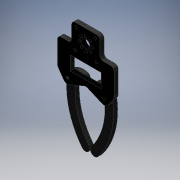
# Autodesk Inventor part: Claw
Saved by Autodesk Inventor 2016 (Build 200138000, 138)
## iProperties
Created: 2015-10-23
Part Number: Claw
Material: Generic
Document SubType Name: Modeling
Designer: alex
Density: 1 g/cm^3
Appearance: Default
Mass: 38.2404 g
Surface Area: 180.646 cm^2
Volume: 38.2404 cm^3
Author: alex
Autodesk Inventor part; units mm, degrees
ref_plane "YZ Plane" through (0, 0, 0) normal (1, 0, 0) x (0, 1, 0)
ref_plane "XZ Plane" through (0, 0, 0) normal (0, 1, 0) x (-1, 0, 0)
ref_plane "XY Plane" through (0, 0, 0) normal (0, 0, 1) x (1, 0, 0)
sketch "Sketch1" plane through (0, 0, 0) normal (0, 1, 0) x (-1, 0, 0)
  line L0 (-20, 14) -> (20, 14)
  line L1 (20, 14) -> (20, -14)
  line L2 (20, -14) -> (-20, -14)
  line L3 (-20, -14) -> (-20, 14)
  line L4 (-20, 14) -> (20, -14) construction
  line L5 (20, 14) -> (-20, -14) construction
  line L6 (-40, -52) -> (40, -52)
  line L7 (40, -52) -> (40, -14)
  line L8 (40, -14) -> (-40, -14)
  line L9 (-40, -14) -> (-40, -52)
  line L10 (-40, -52) -> (40, -14) construction
  line L11 (40, -52) -> (-40, -14) construction
  line L12 (40, -52) -> (28.303, -68.705)
  line L13 (28.303, -68.705) -> (0, -56.6911)
  line L14 (0, -33) -> (0, -82.4656)
  line L15 (-40, -52) -> (-28.303, -68.705)
  line L16 (-28.303, -68.705) -> (0, -56.6911)
  point P0 (0, 0)
  dimension "d0" = 40
  dimension "d1" = 28
  dimension "d2" = 80
  dimension "d3" = 0
  dimension "d4" = 38
  dimension "d5" = 20
  dimension "d6" = 55
  dimension "d7" = 102
  dimension "d8" = 52.1844
  dimension "d9" = 40
  constraints: 34 end point, 4 midpoint, 4 parallel, 2 horizontal, 2 perpendicular, 1 symmetric about line, 1 vertical
  measures "d0" distance of L1.end L2.end
  measures "d1" distance between parallel lines of L2 L0
  measures "d2" distance of L8.end L7.end
  measures "d3" distance between parallel lines of L2 L8
  measures "d4" distance of L6.end L7.end
  measures "d5" distance between parallel lines of L7 L1
  measures "d6" angle of L6 L12
  measures "d7" angle of L13 L12
  measures "d8" distance from line of point (0, 0) L13
  measures "d9" distance from line of L13.end L7
extrude "Extrusion1" add sketch "Sketch1" along normal blind 6
fillet "Fillet1" radius 6 3 edges at (-28.303, 3, -68.705) (28.303, 3, -68.705) (0, 3, -56.6911)
fillet "Fillet2" radius 6 2 edges at (40, 3, -52) (-40, 3, -52)
fillet "Fillet3" radius 5 2 edges at (-40, 3, -14) (40, 3, -14)
fillet "Fillet4" radius 5 2 edges at (-20, 3, -14) (20, 3, -14)
fillet "Fillet5" radius 5 2 edges at (20, 3, 14) (-20, 3, 14)
sketch "Sketch2" plane through (0, 0, 0) normal (0, -1, 0) x (1, 0, 0)
  circle A0 centre (0, -5) radius 6
  line L0 (-15, 14) -> (15, 14) projected
  circle A1 centre (-9, -5.3938) radius 2
  circle A2 centre (-6.0855, -11.6424) radius 2
  circle A3 centre (0.3938, -14) radius 2
  circle A4 centre (6.6424, -11.0855) radius 2
  circle A5 centre (9, -4.6062) radius 2
  circle A6 centre (6.0855, 1.6424) radius 2
  circle A7 centre (-0.3938, 4) radius 2
  circle A8 centre (-6.6424, 1.0855) radius 2
  line L1 (-20, 9) -> (-20, -9) projected
  circle A9 centre (13.5, 8.5) radius 2
  circle A10 centre (-13.5, 8.5) radius 2
  circle A11 centre (15, -20) radius 2
  circle A12 centre (-15, -20) radius 2
  line L2 (20, -9) -> (20, 9) projected
  line L3 (22, -29.2092) -> (-22, -29.2092)
  line L4 (-22, -29.2092) -> (-22, -49.2092)
  line L5 (-22, -49.2092) -> (22, -49.2092)
  line L6 (22, -49.2092) -> (22, -29.2092)
  line L7 (-40, -50.1082) -> (-40, -19) projected
  arc A13 (2.3444, -57.6862) -> (-2.3444, -57.6862) centre (0, -63.2092) ccw projected
  point P0 (0, 0)
  dimension "d17" = 12
  dimension "d18" = 19
  dimension "d19" = 4
  dimension "d22" = 360
  dimension "d24" = 9
  dimension "d25" = 20
  dimension "d26" = 6.6424
  dimension "d29" = 4
  dimension "d35" = 4
  dimension "d36" = 4
  dimension "d37" = 4
  dimension "d40" = 5
  dimension "d41" = 34
  dimension "d42" = 5
  dimension "d43" = 34
  dimension "d44" = 20
  dimension "d45" = 44
  dimension "d46" = 18
  dimension "d47" = 14
  dimension "d72" = 13.5
  dimension "d73" = 13.5
  dimension "d74" = 13.5
  dimension "d75" = 13.5
  constraints: 13 centre point, 8 end point, 2 parallel, 1 horizontal, 1 perpendicular, 17 other
  measures "d17" diameter of A0
  measures "d18" distance from line of L0 A0.centre
  measures "d19" diameter of A1
  measures "d24" horizontal distance of A0.centre A1.centre
  measures "d25" distance from line of L1 A0.centre
  measures "d26" horizontal distance of A0.centre A8.centre
  measures "d29" diameter of A9
  measures "d35" diameter of A10
  measures "d36" diameter of A11
  measures "d37" diameter of A12
  measures "d40" distance from line of L1 A12.centre
  measures "d41" distance from line of L0 A12.centre
  measures "d42" distance from line of L2 A11.centre
  measures "d43" distance from line of L0 A11.centre
  measures "d44" distance between parallel lines of L5 L3
  measures "d45" distance between parallel lines of L4 L6
  measures "d46" distance between parallel lines of L7 L4
  measures "d47" distance from line of A13.centre L5
  measures "d72" horizontal distance of A0.centre A9.centre
  measures "d73" horizontal distance of A0.centre A9.centre
  measures "d74" horizontal distance of A0.centre A10.centre
  measures "d75" horizontal distance of A10.centre A0.centre
extrude "holes" cut sketch "Sketch2" against normal through all
sketch "Sketch3" plane through (0, 0, 0) normal (0, -1, 0) x (1, 0, 0)
  circle A0 centre (26, -59.2092) radius 2
  circle A1 centre (-26, -59.2092) radius 2
  line L0 (22, -29.2092) -> (22, -49.2092) projected
  line L1 (-22, -49.2092) -> (22, -49.2092) projected
  line L2 (-22, -49.2092) -> (-22, -29.2092) projected
  point P0 (0, 0)
  dimension "d48" = 4
  dimension "d49" = 4
  dimension "d50" = 4
  dimension "d51" = 10
  dimension "d52" = 10
  dimension "d53" = 4
  constraints: 2 centre point
  measures "d48" diameter of A0
  measures "d49" diameter of A1
  measures "d50" distance from line of L0 A0.centre
  measures "d51" distance from line of L1 A0.centre
  measures "d52" distance from line of L1 A1.centre
  measures "d53" distance from line of L2 A1.centre
extrude "Extrusion3" cut sketch "Sketch3" against normal through all
sketch "Sketch4" plane through (0, 6, 0) normal (0, 1, 0) x (1, 0, 0)
  line L0 (0, 5.2258) -> (0, 78.3364)
  line L1 (40, 19) -> (40, 50.1082) projected
  arc A0 (25.7862, 59.4415) -> (6.4564, 137.007) centre (-72.0839, 76.243) ccw construction
  arc A1 (31.6836, 58.4291) -> (11.189, 140.6685) centre (-72.0839, 76.243) ccw
  arc A2 (19.8888, 60.454) -> (1.7238, 133.3455) centre (-72.0839, 76.243) ccw
  arc A3 (19.8888, 60.454) -> (31.6836, 58.4291) centre (25.7862, 59.4415) ccw
  arc A4 (11.189, 140.6685) -> (1.7238, 133.3455) centre (6.4564, 137.007) ccw
  arc A5 (-11.189, 140.6685) -> (-31.6836, 58.4291) centre (72.0839, 76.243) ccw
  arc A6 (-1.7238, 133.3455) -> (-19.8888, 60.454) centre (72.0839, 76.243) ccw
  arc A7 (-31.6836, 58.4291) -> (-19.8888, 60.454) centre (-25.7862, 59.4415) ccw
  arc A8 (-1.7238, 133.3455) -> (-11.189, 140.6685) centre (-6.4564, 137.007) ccw
  arc A9 (-25.7862, 59.4415) -> (-11.189, 55.9471) centre (-15.0658, 71.9884) ccw construction
  arc A10 (-29.6632, 54.9041) -> (-9.787, 50.1459) centre (-15.0658, 71.9884) ccw
  arc A11 (-21.9092, 63.979) -> (-12.591, 61.7483) centre (-15.0658, 71.9884) ccw
  arc A12 (-21.9092, 63.979) -> (-29.6632, 54.9041) centre (-25.7862, 59.4415) ccw
  arc A13 (-9.787, 50.1459) -> (-12.591, 61.7483) centre (-11.189, 55.9471) ccw
  arc A14 (9.787, 50.1459) -> (29.6632, 54.9041) centre (15.0658, 71.9884) ccw
  arc A15 (12.591, 61.7483) -> (21.9092, 63.979) centre (15.0658, 71.9884) ccw
  arc A16 (29.6632, 54.9041) -> (21.9092, 63.979) centre (25.7862, 59.4415) ccw
  arc A17 (12.591, 61.7483) -> (9.787, 50.1459) centre (11.189, 55.9471) ccw
  point P0 (0, 0)
  dimension "d56" = 40
  dimension "d57" = 5.9837
  dimension "d58" = 105.2854
  dimension "d59" = 8.3164
  dimension "d60" = 14.2138
  dimension "d61" = 28.811
  dimension "d62" = 11.7644
  dimension "d63" = 48.9574
  dimension "d64" = 60.1201
  dimension "d67" = 5.9682
  dimension "d68" = 22.4712
  dimension "d69" = 49.7871
  dimension "d70" = 51.189
  constraints: 36 point on circle, 18 centre point, 13 symmetric about line, 8 tangent, 2 end point, 1 vertical, 8 other
  measures "d56" distance between parallel lines of L1 L0
  measures "d57" radius of A3
  measures "d58" radius of A1
  measures "d59" distance from line of A1.start L1
  measures "d60" distance from line of A0.start L1
  measures "d61" distance from line of A1.end L1
  measures "d62" distance of L1.end A1.start
  measures "d63" distance of L1.end L0.end
  measures "d64" distance of L1.end L0.start
  measures "d67" radius of A13
  measures "d68" radius of A10
  measures "d69" distance from line of A10.end L1
  measures "d70" distance from line of A9.end L1
extrude "Extrusion4" add sketch "Sketch4" along normal blind 6
fillet "Fillet6" radius 10 2 edges at (20.2646, 9, -62.8257) (-20.2646, 9, -62.8257)
body "Solid1"
